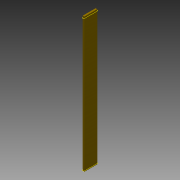
# Autodesk Inventor part: GlassPlate
Saved by Autodesk Inventor 2015 SP1 (Build 190203100, 203)
## iProperties
Created: 2015-08-28
Part Number: GlassPlate
Material: Gold
Document SubType Name: Modeling
Designer: I Rabey
Density: 19.3 g/cm^3
Appearance: Metal 1600F Hot
Author: I Rabey
Autodesk Inventor part; units mm, degrees
ref_plane "YZ Plane" through (0, 0, 0) normal (1, 0, 0) x (0, 1, 0)
ref_plane "XY Plane" through (0, 0, 0) normal (0, 0, 1) x (1, 0, 0)
sketch "Sketch1" plane through (0, 0, 0) normal (1, 0, 0) x (0, 1, 0)
  line L0 (-417.5, -40) -> (417.5, -40)
  line L1 (417.5, -40) -> (417.5, 40)
  line L2 (417.5, 40) -> (-417.5, 40)
  line L3 (-417.5, 40) -> (-417.5, -40)
  line L4 (-417.5, -40) -> (417.5, 40) construction
  line L5 (417.5, -40) -> (-417.5, 40) construction
  point P0 (0, 0)
  dimension "d0" = 835
  dimension "d1" = 80
  constraints: 12 end point, 2 midpoint, 2 parallel, 1 horizontal, 1 perpendicular
  measures "d0" distance of L2.end L1.end
  measures "d1" distance of L2.end L0.start
extrude "Extrusion1" add sketch "Sketch1" along normal blind 10
ref_plane "Work Plane1" through (0, 407.5, 0) normal (0, 1, 0) x (-1, 0, 0)
ref_plane "Work Plane2" through (0, -412.5, 0) normal (0, 1, 0) x (-1, 0, 0)
body "Solid1"
